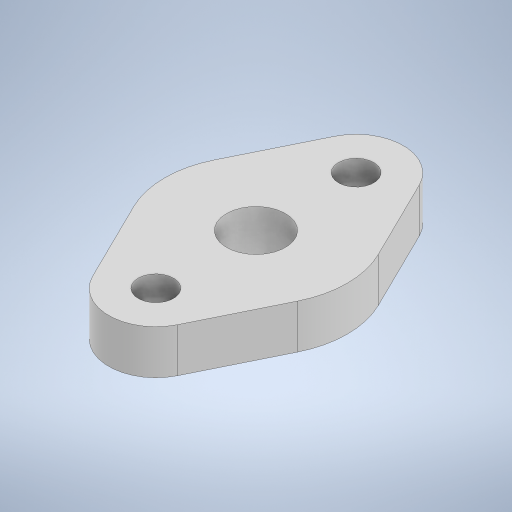
# Autodesk Inventor part: base_obj5
Saved by Autodesk Inventor 2023.2 (Build 272271030, 271C)
## iProperties
Created: 2023-02-25
Part Number: base_obj5
Material: Generic
Document SubType Name: Modeling
Designer: Cris Pat
Density: 1 g/cm^3
Appearance: Default
Author: Cris Pat
Autodesk Inventor part; units mm, degrees
ref_plane "YZ Plane" through (0, 0, 0) normal (1, 0, 0) x (0, 1, 0)
ref_plane "XZ Plane" through (0, 0, 0) normal (0, 1, 0) x (-1, 0, 0)
ref_plane "XY Plane" through (0, 0, 0) normal (0, 0, 1) x (1, 0, 0)
sketch "Sketch1" plane through (0, 0, 0) normal (0, 1, 0) x (-1, 0, 0)
  circle A0 centre (0, -34) radius 6
  circle A1 centre (0, 34) radius 6
  arc A2 (14.5606, -27.3676) -> (14.3587, -41.0588) centre (0, -34) ccw construction
  circle A3 centre (0, 34) radius 16 construction
  circle A4 centre (0, 0) radius 31 construction
  arc A5 (27.82, -13.6765) -> (27.82, 13.6765) centre (0, 0) ccw
  arc A6 (14.3587, 41.0588) -> (0, 50) centre (0, 34) ccw
  line L0 (27.82, 13.6765) -> (14.3587, 41.0588)
  arc A7 (0, -50) -> (14.3587, -41.0588) centre (0, -34) ccw
  line L1 (14.3587, -41.0588) -> (27.82, -13.6765)
  line L2 (0, 34) -> (0, -34) construction
  arc A8 (-27.82, 13.6765) -> (-27.82, -13.6765) centre (0, 0) ccw
  arc A9 (0, 50) -> (-14.3587, 41.0588) centre (0, 34) ccw
  line L3 (-27.82, 13.6765) -> (-14.3587, 41.0588)
  arc A10 (-14.3587, -41.0588) -> (0, -50) centre (0, -34) ccw
  line L4 (-14.3587, -41.0588) -> (-27.82, -13.6765)
  circle A11 centre (0, 0) radius 10
  point P0 (-14.5606, -27.3676)
  dimension "d0" = 12
  dimension "d1" = 68
  dimension "d2" = 34
  dimension "d3" = 32
  dimension "d4" = 62
  dimension "d5" = 20
  constraints: 20 point on circle, 12 centre point, 10 end point, 6 tangent, 5 coincident, 5 symmetric about line, 4 equal radius, 2 vertical alignment, 1 vertical, 3 other
  measures "d0" diameter of A0
  measures "d1" distance of A1.centre A0.centre
  measures "d2" distance of A0.centre point (0, 0)
  measures "d3" diameter of A2
  measures "d4" diameter of A4
  measures "d5" diameter of A11
extrude "Extrusion1" add sketch "Sketch1" along normal mid plane 15
equation "\"d2\" = 0.5 * d1"
body "Solid1"
